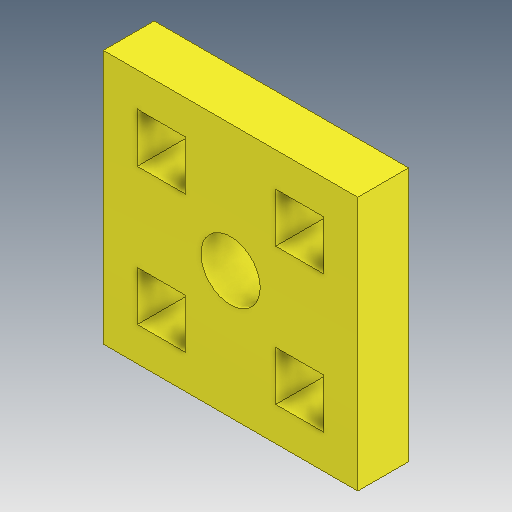
# Autodesk Inventor part: motor_top
Saved by Autodesk Inventor 2020 (Build 240168000, 168)
## iProperties
Created: 2021-05-10
Part Number: motor_top
Material: Generic
Document SubType Name: Modeling
Designer: Hsu Daniel
Density: 1 g/cm^3
Appearance: Canary
Author: Hsu Daniel
Autodesk Inventor part; units mm, degrees
ref_plane "YZ Plane" through (0, 0, 0) normal (1, 0, 0) x (0, 1, 0)
ref_plane "XZ Plane" through (0, 0, 0) normal (0, 1, 0) x (-1, 0, 0)
ref_plane "XY Plane" through (0, 0, 0) normal (0, 0, 1) x (1, 0, 0)
sketch "Sketch1" plane through (0, 0, 0) normal (0, 0, 1) x (1, 0, 0)
  line L0 (-7.5, -7.5) -> (7.5, -7.5)
  line L1 (7.5, -7.5) -> (7.5, 7.5)
  line L2 (7.5, 7.5) -> (-7.5, 7.5)
  line L3 (-7.5, 7.5) -> (-7.5, -7.5)
  line L4 (-7.5, -7.5) -> (7.5, 7.5) construction
  line L5 (7.5, -7.5) -> (-7.5, 7.5) construction
  line L6 (-5.5, 2.58) -> (-2.66, 2.58)
  line L7 (-2.66, 2.58) -> (-2.66, 5.5)
  line L8 (-2.66, 5.5) -> (-5.5, 5.5)
  line L9 (-5.5, 5.5) -> (-5.5, 2.58)
  line L10 (0, 0) -> (0, 4.08) construction
  line L11 (0, 0) -> (5.4269, 0) construction
  line L12 (2.66, 2.58) -> (2.66, 5.5)
  line L13 (2.66, 5.5) -> (5.5, 5.5)
  line L14 (5.5, 5.5) -> (5.5, 2.58)
  line L15 (5.5, 2.58) -> (2.66, 2.58)
  line L16 (2.66, -2.58) -> (2.66, -5.5)
  line L17 (5.5, -2.58) -> (2.66, -2.58)
  line L18 (5.5, -5.5) -> (5.5, -2.58)
  line L19 (2.66, -5.5) -> (5.5, -5.5)
  line L20 (-5.5, -2.58) -> (-2.66, -2.58)
  line L21 (-2.66, -5.5) -> (-5.5, -5.5)
  line L22 (-5.5, -5.5) -> (-5.5, -2.58)
  line L23 (-2.66, -2.58) -> (-2.66, -5.5)
  circle A0 centre (0, 0) radius 1.75
  dimension "d2" = 15
  dimension "d4" = 2.84
  dimension "d5" = 2.92
  dimension "d6" = 2
  dimension "d7" = 2
  dimension "d8" = 3.5
  constraints: 48 end point, 12 symmetric about line, 4 parallel, 3 coincident, 3 horizontal, 3 midpoint, 3 perpendicular, 1 centre point, 1 vertical
  measures "d2" distance of L2.end L1.end
  measures "d4" distance of L8.end L7.end
  measures "d5" distance of L6.end L7.end
  measures "d6" distance between parallel lines of L2 L8
  measures "d7" distance between parallel lines of L3 L9
  measures "d8" diameter of A0
extrude "Extrusion1" add sketch "Sketch1" along normal blind 3
equation "\"d6\" = d7"
equation "\"d8\" = stickL"
equation "\"thick\" = 0.5"
equation "\"lrlr\" = 19"
equation "\"lrmid\" = 19.9"
equation "\"lrdepth\" = 3.3"
equation "\"mlr\" = 16.6"
equation "\"mmid\" = 24.7"
equation "\"mdepth\" = 4.5"
equation "\"lrltotal\" = 126.6"
equation "\"mltotal\" = 126.6"
equation "\"lrbetween\" = 52.1"
equation "\"mbetween\" = 49.5"
equation "\"toler\" = 1"
equation "\"tight\" = 0.08"
equation "\"stuckw\" = 6"
equation "\"sidewallL\" = 132.6"
equation "\"heaterH\" = 117.3"
equation "\"stickL\" = 3.5"
equation "\"wireH\" = 25"
body "Solid1"
